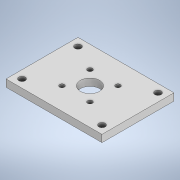
# Autodesk Inventor part: MotorBasePlate
Saved by Autodesk Inventor 2022.1 (Build 261234020, 234B)
## iProperties
Created: 2022-10-16
Part Number: MotorBasePlate
Material: Generic
Document SubType Name: Modeling
Designer: Alexander
Density: 1 g/cm^3
Appearance: Default
Author: Alexander
Autodesk Inventor part; units mm, degrees
ref_plane "YZ Plane" through (0, 0, 0) normal (1, 0, 0) x (0, 1, 0)
ref_plane "XZ Plane" through (0, 0, 0) normal (0, 1, 0) x (-1, 0, 0)
ref_plane "XY Plane" through (0, 0, 0) normal (0, 0, 1) x (1, 0, 0)
sketch "Sketch1" plane through (0, 0, 0) normal (0, 1, 0) x (-1, 0, 0)
  line L0 (0, 0) -> (114.8965, 0) construction
  line L1 (114.8965, 0) -> (114.8965, -52.636) construction
  line L2 (114.8965, -52.636) -> (0, -52.636) construction
  line L3 (0, -52.636) -> (0, 0) construction
  line L4 (81.8737, -2.7526) -> (21.8737, -2.7526)
  line L5 (21.8737, -2.7526) -> (21.8737, -47.7526)
  line L6 (21.8737, -47.7526) -> (81.8737, -47.7526)
  line L7 (81.8737, -47.7526) -> (81.8737, -2.7526)
  circle A0 centre (76.8737, -7.7526) radius 2
  circle A1 centre (51.8737, -25.2526) radius 6
  circle A2 centre (26.8737, -7.7526) radius 2
  circle A3 centre (76.8737, -42.7526) radius 2
  circle A4 centre (26.8737, -42.7526) radius 2
  circle A5 centre (43.1237, -16.5026) radius 1.5
  circle A6 centre (43.1237, -34.0026) radius 1.5
  circle A7 centre (60.6237, -34.0026) radius 1.5
  circle A8 centre (60.6237, -16.5026) radius 1.5
  point P0 (51.8737, -47.7526)
  dimension "d1" = 60
  dimension "d4" = 45
  dimension "d5" = 4
  dimension "d6" = 5
  dimension "d7" = 5
  dimension "d9" = 12
  dimension "d10" = 22.5
  dimension "d11" = 30
  dimension "d16" = 50
  dimension "d19" = 35
  dimension "d37" = 3
  dimension "d49" = 360
  dimension "d52" = 17.5
  constraints: 9 centre point, 8 end point, 2 horizontal, 2 parallel, 1 midpoint, 1 perpendicular, 1 vertical, 17 other
  measures "d1" distance of L4.start L4.end
  measures "d4" distance of L6.end L4.start
  measures "d5" diameter of A0
  measures "d6" distance from line of L7 A0.centre
  measures "d7" distance from line of L4 A0.centre
  measures "d9" diameter of A1
  measures "d10" distance of point (51.874, -47.753) A1.centre
  measures "d11" distance from line of L7 A1.centre
  measures "d16" distance of A0.centre A2.centre
  measures "d19" distance of A0.centre A3.centre
  measures "d37" diameter of A5
  measures "d52" distance of A6.centre A5.centre
extrude "Extrusion1" add sketch "Sketch1" along normal blind 4.5
body "Solid1"
